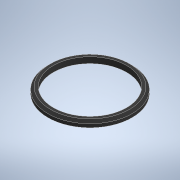
# Autodesk Inventor part: Резина
Saved by Autodesk Inventor 2021 (Build 250183000, 183)
## iProperties
Created: 2020-12-19
Part Number: Резина
Material: Резина
Document SubType Name: Modeling
Designer: Тимоха
Mass: 107.899 g
Surface Area: 334.115 cm^2
Volume: 116.021 cm^3
Density: 0.93 g/cm^3
Appearance: Резина — черная
Author: Тимоха
Autodesk Inventor part; units mm, degrees
ref_plane "YZ Plane" through (0, 0, 0) normal (1, 0, 0) x (0, 1, 0)
ref_plane "XZ Plane" through (0, 0, 0) normal (0, 1, 0) x (-1, 0, 0)
ref_plane "XY Plane" through (0, 0, 0) normal (0, 0, 1) x (1, 0, 0)
sketch "Эскиз1" plane through (0, 0, 0) normal (0, 0, 1) x (1, 0, 0)
  line L0 (0, 0) -> (92.5, 0)
  line L1 (0, 0) -> (100, 0)
  line L2 (100, 0) -> (106.254, -6.254)
  line L3 (106.254, -6.254) -> (106.254, -15)
  line L4 (106.254, -15) -> (92.5, -15)
  line L5 (92.5, -15) -> (92.5, 0)
  line L6 (0, 0) -> (0, -9.5389)
  dimension "d0" = 92.5
  dimension "d1" = 100
  dimension "d2" = 135
  dimension "d3" = 15
  constraints: 14 end point, 2 horizontal, 2 perpendicular, 1 point on line, 1 vertical
  measures "d0" distance of L0.start L0.end
  measures "d1" distance of L0.start L1.end
  measures "d2" angle of L1 L2
  measures "d3" distance from line of L0 L3.end
revolve "Вращение1" add sketch "Эскиз1" angle 360 about axis through (0, 0, 0) along (0, -1, 0)
